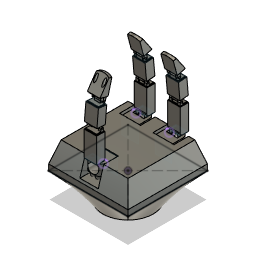
3_finger_gripper_nirmit (Autodesk Fusion 360 design; units mm, degrees)
Autodesk Fusion 360 part; units mm, degrees
note: some values were not read from the file. Chosen so that the rebuilt part matches the saved one: which face or edge a step refers to.
(part 1 of 2)
sketch "Sketch1" plane through (0, 0, 0) normal (0, 1, 0) x (1, 0, 0) in component "base v7"
  circle A0 centre (0, 0) radius 30
  dimension "d3_1" = 60
  constraint coincident A0.centre origin
  measures "d3_1" diameter of A0
ref_plane "WorkPlane1" through (0, 30, 0) normal (0, 1, 0) x (0, 0, 1) in component "base v7"
sketch "Sketch2" plane through (0, 30, 0) normal (0, 1, 0) x (1, 0, 0) in component "base v7"
  line L0 (47.5, 47.5) -> (-47.5, 47.5)
  line L1 (-47.5, 47.5) -> (-47.5, -47.5)
  line L2 (-47.5, -47.5) -> (47.5, -47.5)
  line L3 (47.5, -47.5) -> (47.5, 47.5)
  line L4 (47.5, 47.5) -> (-47.5, -47.5) construction
  line L5 (-47.5, 47.5) -> (47.5, -47.5) construction
  dimension "d6_1" = 95
  dimension "d7_1" = 95
  constraint horizontal L0
  constraint perpendicular L0 L1
  constraint parallel L0 L2
  constraint parallel L1 L3
  constraint coincident L4 origin
  constraint coincident L5 origin
  measures "d6_1" distance of L1.end L2.end
  measures "d7_1" distance of L0.start L2.end
loft "Loft1" add profiles "Sketch1", "Sketch2" section 1 section 2 makes body 1 in component "base v7"
ref_plane "WorkPlane2" through (0, 37, 0) normal (0, 1, 0) x (0, 0, 1) in component "base v7"
sketch "Sketch3" plane through (0, 37, 0) normal (0, 1, 0) x (1, 0, 0) in component "base v7"
  line L0 (47.5, -47.5) -> (-47.5, -47.5)
  line L1 (-47.5, -47.5) -> (-47.5, 47.5)
  line L2 (-47.5, 47.5) -> (47.5, 47.5)
  line L3 (47.5, 47.5) -> (47.5, -47.5)
  line L4 (47.5, -47.5) -> (-47.5, 47.5) construction
  line L5 (-47.5, -47.5) -> (47.5, 47.5) construction
  line L6 (47.5, 47.5) -> (-47.5, 47.5)
  line L7 (47.5, -47.5) -> (47.5, 47.5)
  constraint horizontal L0
  constraint perpendicular L0 L1
  constraint parallel L0 L2
  constraint parallel L1 L3
  constraint coincident L4 origin
  constraint coincident L5 origin
  constraint equal L2 L6
  constraint equal L3 L7
loft "Loft2" add profiles "Sketch2", "Sketch3" section 1 section 2 bodies 1 in component "base v7"
ref_plane "WorkPlane3" through (0, 62, 0) normal (0, 1, 0) x (0, 0, 1) in component "base v7"
sketch "Sketch4" plane through (0, 62, 0) normal (0, 1, 0) x (1, 0, 0) in component "base v7"
  line L0 (40, -40) -> (-40, -40)
  line L1 (-40, -40) -> (-40, 40)
  line L2 (-40, 40) -> (40, 40)
  line L3 (40, 40) -> (40, -40)
  line L4 (40, -40) -> (-40, 40) construction
  line L5 (-40, -40) -> (40, 40) construction
  dimension "d13_1" = 80
  dimension "d14_1" = 80
  constraint horizontal L0
  constraint perpendicular L0 L1
  constraint parallel L0 L2
  constraint parallel L1 L3
  constraint coincident L4 origin
  constraint coincident L5 origin
  measures "d13_1" distance of L1.end L2.end
  measures "d14_1" distance of L0.end L1.end
loft "Loft3" add profiles "Sketch4" section 1 face at (-15.8333, 37, -15.8333) section 2 on bodies 1 bodies 1 in component "base v7"
sketch "Sketch5" plane through (0, 16.1284, 53.7615) normal (0, 0.287348, 0.957826) x (1, 0, 0) in component "base v7"
  line L0 (-47.5, 21.7905) -> (47.5, 21.7905)
  line L1 (47.5, 21.7905) -> (40, 47.8913)
  line L2 (40, 47.8913) -> (-40, 47.8913)
  line L3 (-40, 47.8913) -> (-47.5, 21.7905)
  line L4 (-11, 47.8913) -> (11, 47.8913)
  line L5 (11, 47.8913) -> (11, 25.8913)
  line L6 (11, 25.8913) -> (-11, 25.8913)
  line L7 (-11, 25.8913) -> (-11, 47.8913)
  dimension "d17" = 22
  dimension "d18" = 22
  dimension "d20" = 29
  constraint horizontal L4
  constraint vertical L5
  constraint horizontal L6
  constraint vertical L7
  constraint coincident L2 L4.start
  measures "d17" distance of L4.end L5.end
  measures "d18" distance of L4.start L4.end
  measures "d20" distance of L1.end L5
ref_plane "WorkPlane4" through (0, 33.5, 22.5) normal (0, 0, 1) x (1, 0, 0) in component "base v7"
sketch "Sketch6" plane through (0, 33.5, 22.5) normal (0, 0, 1) x (1, 0, 0) in component "base v7"
  line L0 (-11, 28.5) -> (11, 28.5)
  line L1 (11, 28.5) -> (11, 6.5)
  line L2 (11, 6.5) -> (-11, 6.5)
  line L3 (-11, 6.5) -> (-11, 28.5)
  point P0 (-11, 28.5)
  point P1 (40, 28.5)
  dimension "d23" = 22
  dimension "d24" = 22
  dimension "d25" = 29
  constraint horizontal L0
  constraint vertical L1
  constraint horizontal L2
  constraint vertical L3
  constraint coincident L0 P0
  measures "d23" distance of P0 L2.end
  measures "d24" distance of P0 L0.end
  measures "d25" distance of L1 P1
extrude "Extrude1" cut sketch "Sketch6" along normal through all bodies 1 in component "base v7"
sketch "Sketch7" plane through (0, 0, 22.5) normal (0, 0, 1) x (1, 0, 0) in component "base v7"
  line L0 (-11, 40) -> (11, 40)
  line L1 (11, 40) -> (11, 62)
  line L2 (11, 62) -> (-11, 62)
  line L3 (-11, 62) -> (-11, 40)
  circle A0 centre (0, 51) radius 1.5
  dimension "d29" = 3
  dimension "d30" = 11
  dimension "d31" = 11
  measures "d29" diameter of A0
  measures "d30" distance of L2 A0.centre
  measures "d31" distance of L1 A0.centre
extrude "Extrude2" cut sketch "Sketch7" against normal blind 3 contours A0 bodies 1 in component "base v7"
ref_plane "WorkPlane5" through (0, 33.5, -22.5) normal (0, 0, -1) x (-1, 0, 0) in component "base v7"
sketch "Sketch8" plane through (0, 33.5, -22.5) normal (0, 0, -1) x (1, 0, 0) in component "base v7"
  line L0 (32.5, -28.5) -> (7.5, -28.5)
  line L1 (7.5, -28.5) -> (7.5, -6.5)
  line L2 (7.5, -6.5) -> (32.5, -6.5)
  line L3 (32.5, -6.5) -> (32.5, -28.5)
  line L4 (-7.5, -28.5) -> (-32.5, -28.5)
  line L5 (-32.5, -28.5) -> (-32.5, -6.5)
  line L6 (-32.5, -6.5) -> (-7.5, -6.5)
  line L7 (-7.5, -6.5) -> (-7.5, -28.5)
  line L8 (-40, -28.5) -> (40, -28.5)
  dimension "d35" = 22
  dimension "d36" = 25
  dimension "d37" = 22
  dimension "d38" = 25
  dimension "d42" = 7.5
  dimension "d43" = 7.5
  constraint horizontal L0
  constraint vertical L1
  constraint horizontal L2
  constraint vertical L3
  constraint horizontal L4
  constraint vertical L5
  constraint horizontal L6
  constraint vertical L7
  constraint coincident L0.start L8
  constraint coincident L4.start L8
  measures "d35" distance of L0.start L2.end
  measures "d36" distance of L0.start L0.end
  measures "d37" distance of L4.end L5.end
  measures "d38" distance of L4.start L4.end
  measures "d42" distance of L3 L8.end
  measures "d43" distance of L5 L8.start
extrude "Extrude3" cut sketch "Sketch8" along normal through all bodies 1 in component "base v7"
sketch "Sketch9" plane through (0, 0, -22.5) normal (0, 0, -1) x (-1, 0, 0) in component "base v7"
  line L0 (-7.5, 62) -> (-32.5, 62)
  line L1 (-32.5, 62) -> (-32.5, 40)
  line L2 (-32.5, 40) -> (-7.5, 40)
  line L3 (-7.5, 40) -> (-7.5, 62)
  circle A0 centre (-20, 51) radius 1.5
  circle A1 centre (20, 51) radius 1.5
  line L4 (7.5, 40) -> (7.5, 62)
  line L5 (7.5, 62) -> (32.5, 62)
  dimension "d45" = 3
  dimension "d46" = 11
  dimension "d47" = 12.5
  dimension "d48" = 3
  dimension "d49" = 12.5
  dimension "d50" = 11
  measures "d45" diameter of A0
  measures "d46" distance of L0 A0.centre
  measures "d47" distance of L1 A0.centre
  measures "d48" diameter of A1
  measures "d49" distance of A1.centre L4
  measures "d50" distance of A1.centre L5
extrude "Extrude4" cut sketch "Sketch9" against normal blind 3 contours A0 | A1 bodies 1 in component "base v7"
sketch "Sketch1 (2)" plane through (0, 0, 0) normal (1, 0, 0) x (0, 0, -1) in component "top v5"
  line L0 (0, 0) -> (20, 0)
  line L1 (20, 0) -> (20, 10)
  line L2 (20, 10) -> (0, 3)
  line L3 (0, 3) -> (0, 0)
  dimension "d5_3" = 20
  dimension "d6_3" = 10
  dimension "d7_3" = 3
  constraint coincident L0.start L3.end
  constraint horizontal L0
  constraint perpendicular L0 L1
  constraint perpendicular L0 L3
  measures "d5_3" distance of L0.start L0.end
  measures "d6_3" distance of L0.end L1.end
  measures "d7_3" distance of L2.end L0.start
extrude "Extrude1'" add sketch "Sketch1 (2)" along normal blind 15 separate body makes body 2 in component "top v5"
sketch "Sketch2 (2)" plane through (15, 0, 0) normal (1, 0, 0) x (0, 0, -1) in component "top v5"
  line L0 (0, 3) -> (0, 0)
  line L1 (0, 0) -> (20, 0)
  line L2 (20, 0) -> (20, 10)
  line L3 (20, 10) -> (0, 3)
ref_plane "WorkPlane1" through (7.5, 5, -21) normal (0, 0, -1) x (0, 1, 0) in component "top v5"
sketch "Sketch3 (2)" plane through (7.5, 5, -21) normal (0, 0, -1) x (1, 0, 0) in component "top v5"
  line L0 (-6.5, 4) -> (6.5, 4)
  line L1 (6.5, 4) -> (6.5, -4)
  line L2 (6.5, -4) -> (-6.5, -4)
  line L3 (-6.5, -4) -> (-6.5, 4)
  line L4 (-6.5, 4) -> (6.5, -4) construction
  line L5 (6.5, 4) -> (-6.5, -4) construction
  dimension "d17_2" = 13
  dimension "d18_2" = 8
  constraint horizontal L0
  constraint perpendicular L0 L1
  constraint parallel L0 L2
  constraint parallel L1 L3
  constraint coincident L4 origin
  constraint coincident L5 origin
  measures "d17_2" distance of L1.end L2.end
  measures "d18_2" distance of L0.start L2.end
extrude "Extrude2'" add sketch "Sketch3 (2)" against normal blind 1 bodies 2 in component "top v5"
sketch "Sketch4 (2)" plane through (14, 0, 0) normal (1, 0, 0) x (0, 0, -1) in component "top v5"
  line L0 (21, 1) -> (21, 9)
  line L1 (21, 9) -> (20, 9)
  line L2 (20, 9) -> (20, 1)
  line L3 (20, 1) -> (21, 1)
  line L4 (21, 2.5) -> (25, 2.5) construction
  circle A0 centre (25, 2.5) radius 1.5
  line L5 (0, 0) -> (20, 0)
  circle A1 centre (25, 2.5) radius 1
  line L6 (21, 4) -> (25, 4)
  line L7 (21, 1) -> (25, 1)
  dimension "d22_1" = 3
  dimension "d24_1" = 4
  dimension "d26_2" = 2
  dimension "d27_1" = 1.5
  constraint coincident L0 L4.start
  constraint perpendicular L0 L4
  constraint coincident L4.end A0.centre
  constraint concentric A0 A1
  constraint coincident L0 L6.start
  constraint perpendicular L0 L6
  constraint tangent A0 L6
  constraint horizontal L7
  constraint tangent A0 L7
  constraint coincident A0 L6.end
  constraint coincident L0.start L3.end
  constraint coincident A0 L7.end
  measures "d22_1" diameter of A0
  measures "d24_1" distance of L4.start L4.end
  measures "d26_2" diameter of A1
  measures "d27_1" distance of L3 L4
extrude "Extrude3'" add sketch "Sketch4 (2)" against normal blind 3 contours L0 A0 L6 L7 | A0 bodies 2 in component "top v5"
sketch "Sketch5 (2)" plane through (1, 0, 0) normal (-1, 0, 0) x (0, 0, 1) in component "top v5"
  line L0 (-21, 9) -> (-21, 1)
  line L1 (-21, 1) -> (-20, 1)
  line L2 (-20, 1) -> (-20, 9)
  line L3 (-20, 9) -> (-21, 9)
  circle A0 centre (-25, 2.5) radius 1.5
  circle A1 centre (-25, 2.5) radius 1
  line L4 (-25, 4) -> (-21, 4)
  line L5 (-21, 1) -> (-25, 1)
  line L6 (-21, 2.5) -> (-25, 2.5) construction
  point P0 (-25, 2.5)
  dimension "d31_1" = 3
  dimension "d32_1" = 2
  dimension "d33_1" = 3
  dimension "d34_1" = 4
  constraint concentric A0 A1
  constraint coincident L0 L4.end
  constraint perpendicular L0 L4
  constraint coincident L0.end L1.start
  constraint perpendicular L0 L5
  constraint coincident A0 L5.end
  constraint tangent A0 L4
  constraint coincident A0 L4.start
  constraint coincident L0 L6.start
  constraint coincident P0 A0.centre
  constraint coincident L6 P0
  measures "d31_1" diameter of A0
  measures "d32_1" diameter of A1
  measures "d33_1" distance of L4 L5
  measures "d34_1" distance of L6.start P0
extrude "Extrude4'" add sketch "Sketch5 (2)" against normal blind 3 contours L0 A0 L4 L5 | A0 bodies 2 in component "top v5"
sketch "Sketch6 (2)" plane through (0, 0, 0) normal (0, -1, 0) x (1, 0, 0) in component "top v5"
  line L0 (0, 0) -> (0, -20)
  line L1 (0, -20) -> (15, -20)
  line L2 (15, -20) -> (15, 0)
  line L3 (15, 0) -> (0, 0)
sketch "Sketch7 (2)" plane through (0, 0, -21) normal (0, 0, -1) x (-1, 0, 0) in component "top v5"
  line L0 (-4, 4) -> (-1, 4)
  line L1 (-1, 4) -> (-1, 9)
  line L2 (-1, 9) -> (-14, 9)
  line L3 (-14, 9) -> (-14, 4)
  line L4 (-14, 4) -> (-11, 4)
  line L5 (-11, 4) -> (-11, 1)
  line L6 (-11, 1) -> (-4, 1)
  line L7 (-4, 1) -> (-4, 4)
sketch "Sketch8 (2)" plane through (0, 0, -21) normal (0, 0, -1) x (-1, 0, 0) in component "top v5"
sketch "Sketch9 (2)" plane through (0, 0, 0) normal (0, 0, 1) x (1, 0, 0) in component "top v5"
  line L0 (0, 3) -> (0, 0)
  line L1 (0, 0) -> (15, 0)
  line L2 (15, 0) -> (15, 3)
  line L3 (15, 3) -> (0, 3)
  circle A0 centre (2.5, 5.5) radius 1.5
  line L4 (0, 10) -> (0, 3)
  line L5 (7.5, 3) -> (7.5, 9.6608) construction
  circle A1 centre (12.5, 5.5) radius 1.5
  dimension "d41" = 3
  dimension "d42_1" = 2.5
  dimension "d43_1" = 2.5
  constraint midpoint L3 L5.start
  constraint perpendicular L3 L5
  constraint symmetric A0 L5 A1
  measures "d41" diameter of A0
  measures "d42_1" distance of L3 A0.centre
  measures "d43_1" distance of A0.centre L4
extrude "Extrude5" cut sketch "Sketch9 (2)" against normal blind 15 contours A0 | A1 bodies 2 in component "top v5"
sketch "Sketch10" plane through (0, 0, 0) normal (0, -1, 0) x (1, 0, 0) in component "top v5"
sketch "Sketch11" plane through (0, 0, 0) normal (0, -1, 0) x (1, 0, 0) in component "top v5"
sketch "Sketch12" plane through (0, 0, 0) normal (0, -1, 0) x (1, 0, 0) in component "top v5"
  line L0 (0, 0) -> (0, -20)
  line L1 (0, -20) -> (15, -20)
  line L2 (15, -20) -> (15, 0)
  line L3 (15, 0) -> (0, 0)
  spline S0 degree 5 poles (0, -2) (0.5838, -1.6896) (1.7517, -1.1357) (3.5045, -0.5055) (5.8468, -0.0305) (8.8064, 0.0199) (11.2274, -0.4094) (13.0916, -1.0608) (14.3597, -1.6595) (15, -2) knots 0 0 0 0 0 0 0.2 0.4 0.6 0.8 1 1 1 1 1 1
  line L4 (13.4574, -1.1798) -> (16.5426, -2.8202)
  line L5 (15, -20) -> (15, 0)
  line L6 (-1.4063, -2.7478) -> (1.4063, -1.2522)
  line L7 (0, 0) -> (0, -20)
  line L8 (0, -2) -> (0, 0)
  line L9 (15, 0) -> (15, -2)
  dimension "d46_1" = 62
  dimension "d47_1" = 62
  dimension "d53" = 2
  dimension "d54" = 2
  constraint coincident L0 S0.start
  constraint coincident L2 S0.end
  constraint midpoint S0.end L4
  constraint midpoint S0.start L6
  constraint coincident L0.start L3.end
  constraint coincident L2.end L3.start
  measures "d46_1" angle of L4 L5
  measures "d47_1" angle of L6 L7
  measures "d53" distance of L0.start S0.start
  measures "d54" distance of S0.end L2.end
extrude "Extrude6" cut sketch "Sketch12" against normal through all contours L0 L2 L3 S0 L5 L7 L8 L9 bodies 2 in component "top v5"
sketch "Sketch1 (3)" plane through (0, 0, 0) normal (0, 1, 0) x (1, 0, 0) in component "middle v4"
  line L0 (7.5, -10) -> (-7.5, -10)
  line L1 (-7.5, -10) -> (-7.5, 10)
  line L2 (-7.5, 10) -> (7.5, 10)
  line L3 (7.5, 10) -> (7.5, -10)
  line L4 (7.5, -10) -> (-7.5, 10) construction
  line L5 (-7.5, -10) -> (7.5, 10) construction
  dimension "d4_2" = 15
  dimension "d5_4" = 20
  constraint horizontal L0
  constraint perpendicular L0 L1
  constraint parallel L0 L2
  constraint parallel L1 L3
  constraint coincident L4 origin
  constraint coincident L5 origin
  measures "d4_2" distance of L1.end L2.end
  measures "d5_4" distance of L0.start L2.end
extrude "Extrude1''" add sketch "Sketch1 (3)" along normal blind 10 separate body makes body 3 in component "middle v4"
sketch "Sketch2 (3)" plane through (0, 0, -10) normal (0, 0, -1) x (-1, 0, 0) in component "middle v4"
  line L0 (-7.5, 0) -> (7.5, 0)
  line L1 (7.5, 0) -> (7.5, 10)
  line L2 (7.5, 10) -> (-7.5, 10)
  line L3 (-7.5, 10) -> (-7.5, 0)
sketch "Sketch3 (3)" plane through (0, 0, -10) normal (0, 0, -1) x (-1, 0, 0) in component "middle v4"
  line L0 (-6.5, 9) -> (6.5, 9)
  line L1 (6.5, 9) -> (6.5, 1)
  line L2 (6.5, 1) -> (-6.5, 1)
  line L3 (-6.5, 1) -> (-6.5, 9)
  line L4 (7.5, 10) -> (-7.5, 10)
  line L5 (-7.5, 10) -> (-7.5, 0)
  dimension "d11_1" = 8
  dimension "d12_2" = 13
  dimension "d13_2" = 1
  dimension "d14_2" = 1
  constraint horizontal L0
  constraint vertical L1
  constraint horizontal L2
  constraint vertical L3
  measures "d11_1" distance of L0.end L1.end
  measures "d12_2" distance of L0.start L0.end
  measures "d13_2" distance of L0 L4
  measures "d14_2" distance of L3 L5
extrude "Extrude2''" add sketch "Sketch3 (3)" along normal blind 1 bodies 3 in component "middle v4"
sketch "Sketch4 (3)" plane through (0, 0, -11) normal (0, 0, -1) x (-1, 0, 0) in component "middle v4"
  line L0 (-6.5, 1) -> (6.5, 1)
  line L1 (6.5, 1) -> (6.5, 9)
  line L2 (6.5, 9) -> (-6.5, 9)
  line L3 (-6.5, 9) -> (-6.5, 1)
ref_plane "WorkPlane1" through (0, 5, -10.5) normal (1, 0, 0) x (0, -1, 0) in component "middle v4"
sketch "Sketch5 (3)" plane through (0, 5, -10.5) normal (1, 0, 0) x (0, 0, -1) in component "middle v4"
sketch "Sketch6 (3)" plane through (0, 0, -11) normal (0, 0, -1) x (-1, 0, 0) in component "middle v4"
sketch "Sketch7 (3)" plane through (0, 0, -11) normal (0, 0, -1) x (-1, 0, 0) in component "middle v4"
sketch "Sketch8 (3)" plane through (0, 0, -11) normal (0, 0, -1) x (1, 0, 0) in component "middle v4"
sketch "Sketch9 (3)" plane through (0, 5, -10.5) normal (1, 0, 0) x (0, 0, -1) in component "middle v4"
sketch "Sketch10 (2)" plane through (0, 5, -10.5) normal (1, 0, 0) x (0, 0, -1) in component "middle v4"
sketch "Sketch11 (2)" plane through (0, 5, -10.5) normal (1, 0, 0) x (0, 0, -1) in component "middle v4"
  line L0 (0, 0) -> (0.5, 0) construction
  line L1 (0.5, 0) -> (0.5, -4) construction
  circle A0 centre (3, -2.5) radius 1
  circle A1 centre (3, -2.5) radius 1.5
  line L2 (0.5, -2.5) -> (3, -2.5) construction
  line L3 (0.5, -4) -> (3, -4)
  line L4 (0.5, -1) -> (3, -1)
  line L5 (0.5, -1) -> (0.5, -4)
  dimension "d18_3" = 0.5
  dimension "d19_2" = 4
  dimension "d22_2" = 3
  dimension "d23_1" = 2
  dimension "d25_2" = 2.5
  constraint coincident L0.start origin
  constraint horizontal L0
  constraint perpendicular L0 L1
  constraint concentric A0 A1
  constraint coincident L1 L2.start
  constraint perpendicular L1 L2
  constraint coincident A0.centre A1.centre
  constraint perpendicular L1 L3
  constraint tangent A1 L3
  constraint coincident A1 L3.end
  constraint coincident L1 L4.start
  constraint perpendicular L1 L4
  constraint tangent A1 L4
  constraint coincident A1 L4.end
  measures "d18_3" distance of L0.start L0.end
  measures "d19_2" distance of L0.end L1.end
  measures "d22_2" diameter of A1
  measures "d23_1" diameter of A0
  measures "d25_2" distance of L2.start A0.centre
sketch "Sketch12 (2)" plane through (0, 5, -10.5) normal (1, 0, 0) x (0, 0, -1) in component "middle v4"
extrude "Extrude3''" add sketch "Sketch11 (2)" along normal blind 3.5 and the other way blind 3.5 bodies 3 in component "middle v4"
ref_plane "WorkPlane2" through (0, 5, 0) normal (0, 0, 1) x (1, 0, 0) in component "middle v4"
mirror "Mirror1" about plane through (0, 5, 0) normal (0, 0, 1) of "Extrude2''", "Extrude3''" in component "middle v4"
sketch "Sketch1 (4)" plane through (0, 0, 0) normal (0, 1, 0) x (1, 0, 0) in component "end v6"
  line L0 (7.5, -15) -> (-7.5, -15)
  line L1 (-7.5, -15) -> (-7.5, 15)
  line L2 (-7.5, 15) -> (7.5, 15)
  line L3 (7.5, 15) -> (7.5, -15)
  line L4 (7.5, -15) -> (-7.5, 15) construction
  line L5 (-7.5, -15) -> (7.5, 15) construction
  dimension "d4_3" = 30
  dimension "d5_5" = 15
  constraint horizontal L0
  constraint perpendicular L0 L1
  constraint parallel L0 L2
  constraint parallel L1 L3
  constraint coincident L4 origin
  constraint coincident L5 origin
  measures "d4_3" distance of L0.start L2.end
  measures "d5_5" distance of L0.start L0.end
extrude "Extrude1'''" add sketch "Sketch1 (4)" along normal blind 10 separate body makes body 4 in component "end v6"
sketch "Sketch2 (4)" plane through (0, 0, -15) normal (0, 0, -1) x (-1, 0, 0) in component "end v6"
  line L0 (-7.5, 0) -> (7.5, 0)
  line L1 (7.5, 0) -> (7.5, 10)
  line L2 (7.5, 10) -> (-7.5, 10)
  line L3 (-7.5, 10) -> (-7.5, 0)
  line L4 (-6.5, 9) -> (6.5, 9)
  line L5 (6.5, 9) -> (6.5, 1)
  line L6 (6.5, 1) -> (-6.5, 1)
  line L7 (-6.5, 1) -> (-6.5, 9)
  dimension "d10_1" = 13
  dimension "d11_2" = 8
  dimension "d12_3" = 1
  dimension "d13_3" = 1
  constraint horizontal L4
  constraint vertical L5
  constraint horizontal L6
  constraint vertical L7
  measures "d10_1" distance of L4.start L4.end
  measures "d11_2" distance of L4.end L5.end
  measures "d12_3" distance of L2 L4
  measures "d13_3" distance of L3 L7
extrude "Extrude2'''" add sketch "Sketch2 (4)" along normal blind 1 contours L4 L5 L6 L7 bodies 4 in component "end v6"
ref_plane "WorkPlane1" through (0, 5, -15.5) normal (1, 0, 0) x (0, -1, 0) in component "end v6"
sketch "Sketch3 (4)" plane through (6.5, 0, 0) normal (1, 0, 0) x (0, 0, -1) in component "end v6"
  line L0 (15, 9) -> (15, 1)
  line L1 (15, 1) -> (16, 1)
  line L2 (16, 1) -> (16, 9)
  line L3 (16, 9) -> (15, 9)
  line L4 (16, 1) -> (18.5, 1)
  line L5 (16, 2.5) -> (18.5, 2.5) construction
  circle A0 centre (18.5, 2.5) radius 1.5
  circle A1 centre (18.5, 2.5) radius 1
  line L6 (16, 4) -> (18.5, 4)
  dimension "d20_3" = 2.5
  dimension "d21" = 3
  dimension "d22_3" = 2
  constraint coincident L1.end L2.start
  constraint perpendicular L2 L4
  constraint coincident L2 L5.start
  constraint perpendicular L2 L5
  constraint coincident L5.end A0.centre
  constraint concentric A0 A1
  constraint coincident L2 L6.start
  constraint perpendicular L2 L6
  constraint tangent L4 A0
  constraint tangent A0 L6
  constraint coincident A0 L6.end
  constraint coincident L4.end A0
  measures "d20_3" distance of L5.start L5.end
  measures "d21" diameter of A0
  measures "d22_3" diameter of A1
extrude "Extrude3'''" add sketch "Sketch3 (4)" against normal blind 3 contours L2 L4 A0 L6 | A0 bodies 4 in component "end v6"
mirror "Mirror1'" about plane through (0, 5, -15.5) normal (1, 0, 0) of "Extrude2'''", "Extrude3'''" in component "end v6"
ref_plane "WorkPlane2" through (0, 5, 0) normal (0, 0, 1) x (1, 0, 0) in component "end v6"
mirror "Mirror2" about plane through (0, 5, 0) normal (0, 0, 1) of 13 faces at (3.5, 2.5, -16.5) (4.5, 3.4925, -19.6247) (5.5, 4, -16.8333) (-4.5, 3.5474, -19.5738) (-6.5, 2.5, -16.1667) (-5.5, 4, -16.8333) (1.1667, 7.3333, -16) (6.5, 2.5, -16.1667) (2.1667, 9, -15.3333) (5.5, 1, -16.5) (-3.5, 2.5, -16.5) (5.5, 2.4004, -19.495) (-5.5, 2.4004, -19.495) on bodies 4 in component "end v6"
sketch "Sketch4 (4)" plane through (0, 0, 15) normal (0, 0, 1) x (1, 0, 0) in component "end v6"
  line L0 (6.5, 9) -> (6.5, 1)
  line L1 (6.5, 1) -> (-6.5, 1)
  line L2 (-6.5, 1) -> (-6.5, 9)
  line L3 (-6.5, 9) -> (6.5, 9)
  line L4 (-7.5, 0) -> (7.5, 0)
  line L5 (7.5, 0) -> (7.5, 10)
  line L6 (7.5, 10) -> (-7.5, 10)
  line L7 (-7.5, 10) -> (-7.5, 0)
sketch "Sketch5 (4)" plane through (6.5, 0, 0) normal (1, 0, 0) x (0, 0, -1) in component "end v6"
  circle A0 centre (-18.5, 2.5) radius 1
  line L0 (-16, 9) -> (-16, 4)
  line L1 (-16, 4) -> (-18.5, 4)
  arc A1 (-18.5, 4) -> (-18.5, 1) centre (-18.5, 2.5) ccw
  line L2 (-18.5, 1) -> (-15, 1)
  line L3 (-15, 1) -> (-15, 9)
  line L4 (-15, 9) -> (-16, 9)
sketch "Sketch6 (4)" plane through (0, 0, 16) normal (0, 0, 1) x (1, 0, 0) in component "end v6"
  line L0 (-3.5, 4) -> (-3.5, 1)
  line L1 (-3.5, 1) -> (3.5, 1)
  line L2 (3.5, 1) -> (3.5, 4)
  line L3 (3.5, 4) -> (6.5, 4)
  line L4 (6.5, 4) -> (6.5, 9)
  line L5 (6.5, 9) -> (-6.5, 9)
  line L6 (-6.5, 9) -> (-6.5, 4)
  line L7 (-6.5, 4) -> (-3.5, 4)
fillet "Fillet1" radius 3 1 edges at (0, 0, 15) on bodies 4 in component "end v6"
sketch "Sketch1 (5)" plane through (0, 0, 0) normal (1, 0, 0) x (0, 0, -1) in component "turner v14"
  line L0 (10, -10) -> (-10, -10)
  line L1 (-10, -10) -> (-10, 10)
  line L2 (-10, 10) -> (10, 10)
  line L3 (10, 10) -> (10, -10)
  line L4 (10, -10) -> (-10, 10) construction
  line L5 (-10, -10) -> (10, 10) construction
  dimension "d4_4" = 20
  dimension "d5_6" = 20
  constraint horizontal L0
  constraint perpendicular L0 L1
  constraint parallel L0 L2
  constraint parallel L1 L3
  constraint coincident L4 origin
  constraint coincident L5 origin
  measures "d4_4" distance of L0.start L2.end
  measures "d5_6" distance of L0.start L0.end
extrude "Extrude1''''" add sketch "Sketch1 (5)" along normal blind 20 separate body makes body 5 in component "turner v14"
sketch "Sketch2 (5)" plane through (0, 0, -10) normal (0, 0, -1) x (-1, 0, 0) in component "turner v14"
  line L0 (0, -10) -> (0, 10)
  line L1 (0, 10) -> (-20, 10)
  line L2 (-20, 10) -> (-20, -10)
  line L3 (-20, -10) -> (0, -10)
  line L4 (-10, 10) -> (-3.5, 10)
  line L5 (-3.5, 10) -> (-3.5, 3.5)
  line L6 (-10, 10) -> (-10, 4.4853) construction
  line L7 (-10, 10) -> (-16.5, 10)
  line L8 (-16.5, 10) -> (-16.5, 3.5)
  arc A0 (-16.5, 3.5) -> (-3.5, 3.5) centre (-10, 3.5) ccw
  dimension "d12_4" = 6.5
  dimension "d13_4" = 6.5
  constraint midpoint L1 L4.start
  constraint parallel L1 L4
  constraint perpendicular L4 L5
  constraint perpendicular L1 L6
  constraint symmetric L4.start L6 L7.start
  constraint symmetric L4.end L6 L7.end
  constraint symmetric L5.end L6 L8.end
  constraint tangent L5 A0
  measures "d12_4" distance of L4.start L4.end
  measures "d13_4" distance of L4.end L5.end
extrude "Extrude2''''" cut sketch "Sketch2 (5)" against normal blind 10 contours L1 L4 L5 L7 L8 A0 bodies 5 in component "turner v14"
sketch "Sketch3 (5)" plane through (3.5, 0, 0) normal (1, 0, 0) x (0, 0, -1) in component "turner v14"
  line L0 (10, 3.5) -> (10, 10)
  line L1 (10, 10) -> (0, 10)
  line L2 (0, 10) -> (0, 3.5)
  line L3 (0, 3.5) -> (10, 3.5)
  line L4 (5, 3.5) -> (5, 7.5) construction
  circle A0 centre (5, 7.5) radius 1
  dimension "d20_4" = 4
  dimension "d22_4" = 5
  dimension "d23_2" = 2
  constraint coincident L3 L4.start
  constraint perpendicular L3 L4
  constraint coincident L4.end A0.centre
  measures "d20_4" distance of L4.start L4.end
  measures "d22_4" distance of L0 L4
  measures "d23_2" diameter of A0
extrude "Extrude3''''" add sketch "Sketch3 (5)" along normal up to surface (13 mm away) contours A0 bodies 5 in component "turner v14"
sketch "Sketch4 (5)" plane through (0, 0, 10) normal (0, 0, 1) x (1, 0, 0) in component "turner v14"
  line L0 (0, 10) -> (0, -10)
  line L1 (0, -10) -> (20, -10)
  line L2 (20, -10) -> (20, 10)
  line L3 (20, 10) -> (0, 10)
sketch "Sketch5 (5)" plane through (0, 0, 10) normal (0, 0, 1) x (1, 0, 0) in component "turner v14"
  circle A0 centre (10, 0) radius 1.5
  line L0 (20, 10) -> (0, 10)
  line L1 (20, -10) -> (20, 10)
  dimension "d28_3" = 3
  dimension "d29_5" = 10
  dimension "d30_4" = 10
  measures "d28_3" diameter of A0
  measures "d29_5" distance of A0.centre L0
  measures "d30_4" distance of A0.centre L1
extrude "Extrude4''" add sketch "Sketch5 (5)" along normal blind 3 bodies 5 in component "turner v14"
fillet "Fillet1'" radius 7 1 edges at (10, -10, -10) on bodies 5 in component "turner v14"
fillet "Fillet2" radius 7 3 edges at (20, -10, 3.5) (20, -7.9497, -7.9497) (20, 3.5, -10) on bodies 5 in component "turner v14"
fillet "Fillet3" radius 7 3 edges at (0, 3.5, -10) (0, -7.9497, -7.9497) (0, -10, 3.5) on bodies 5 in component "turner v14"
sketch "Sketch1 (6)" plane through (0, 0, 0) normal (1, 0, 0) x (0, 0, -1) in component "top v5 (1)"
  line L0 (0, 0) -> (20, 0)
  line L1 (20, 0) -> (20, 10)
  line L2 (20, 10) -> (0, 3)
  line L3 (0, 3) -> (0, 0)
  dimension "d5_8" = 20
  dimension "d6_7" = 10
  dimension "d7_7" = 3
  constraint coincident L0.start L3.end
  constraint horizontal L0
  constraint perpendicular L0 L1
  constraint perpendicular L0 L3
  measures "d5_8" distance of L0.start L0.end
  measures "d6_7" distance of L0.end L1.end
  measures "d7_7" distance of L2.end L0.start
extrude "Extrude1'''''" add sketch "Sketch1 (6)" along normal blind 15 separate body makes body 6 in component "top v5 (1)"
sketch "Sketch2 (6)" plane through (15, 0, 0) normal (1, 0, 0) x (0, 0, -1) in component "top v5 (1)"
  line L0 (0, 3) -> (0, 0)
  line L1 (0, 0) -> (20, 0)
  line L2 (20, 0) -> (20, 10)
  line L3 (20, 10) -> (0, 3)
ref_plane "WorkPlane1" through (7.5, 5, -21) normal (0, 0, -1) x (0, 1, 0) in component "top v5 (1)"
sketch "Sketch3 (6)" plane through (7.5, 5, -21) normal (0, 0, -1) x (1, 0, 0) in component "top v5 (1)"
  line L0 (-6.5, 4) -> (6.5, 4)
  line L1 (6.5, 4) -> (6.5, -4)
  line L2 (6.5, -4) -> (-6.5, -4)
  line L3 (-6.5, -4) -> (-6.5, 4)
  line L4 (-6.5, 4) -> (6.5, -4) construction
  line L5 (6.5, 4) -> (-6.5, -4) construction
  dimension "d17_4" = 13
  dimension "d18_5" = 8
  constraint horizontal L0
  constraint perpendicular L0 L1
  constraint parallel L0 L2
  constraint parallel L1 L3
  constraint coincident L4 origin
  constraint coincident L5 origin
  measures "d17_4" distance of L1.end L2.end
  measures "d18_5" distance of L0.start L2.end
extrude "Extrude2'''''" add sketch "Sketch3 (6)" against normal blind 1 bodies 6 in component "top v5 (1)"
sketch "Sketch4 (6)" plane through (14, 0, 0) normal (1, 0, 0) x (0, 0, -1) in component "top v5 (1)"
  line L0 (21, 1) -> (21, 9)
  line L1 (21, 9) -> (20, 9)
  line L2 (20, 9) -> (20, 1)
  line L3 (20, 1) -> (21, 1)
  line L4 (21, 2.5) -> (25, 2.5) construction
  circle A0 centre (25, 2.5) radius 1.5
  line L5 (0, 0) -> (20, 0)
  circle A1 centre (25, 2.5) radius 1
  line L6 (21, 4) -> (25, 4)
  line L7 (21, 1) -> (25, 1)
  dimension "d22_5" = 3
  dimension "d24_4" = 4
  dimension "d26_5" = 2
  dimension "d27_5" = 1.5
  constraint coincident L0 L4.start
  constraint perpendicular L0 L4
  constraint coincident L4.end A0.centre
  constraint concentric A0 A1
  constraint coincident L0 L6.start
  constraint perpendicular L0 L6
  constraint tangent A0 L6
  constraint horizontal L7
  constraint tangent A0 L7
  constraint coincident A0 L6.end
  constraint coincident L0.start L3.end
  constraint coincident A0 L7.end
  measures "d22_5" diameter of A0
  measures "d24_4" distance of L4.start L4.end
  measures "d26_5" diameter of A1
  measures "d27_5" distance of L3 L4
extrude "Extrude3'''''" add sketch "Sketch4 (6)" against normal blind 3 contours L0 A0 L6 L7 | A0 bodies 6 in component "top v5 (1)"
sketch "Sketch5 (6)" plane through (1, 0, 0) normal (-1, 0, 0) x (0, 0, 1) in component "top v5 (1)"
  line L0 (-21, 9) -> (-21, 1)
  line L1 (-21, 1) -> (-20, 1)
  line L2 (-20, 1) -> (-20, 9)
  line L3 (-20, 9) -> (-21, 9)
  circle A0 centre (-25, 2.5) radius 1.5
  circle A1 centre (-25, 2.5) radius 1
  line L4 (-25, 4) -> (-21, 4)
  line L5 (-21, 1) -> (-25, 1)
  line L6 (-21, 2.5) -> (-25, 2.5) construction
  point P0 (-25, 2.5)
  dimension "d31_5" = 3
  dimension "d32_5" = 2
  dimension "d33_2" = 3
  dimension "d34_2" = 4
  constraint concentric A0 A1
  constraint coincident L0 L4.end
  constraint perpendicular L0 L4
  constraint coincident L0.end L1.start
  constraint perpendicular L0 L5
  constraint coincident A0 L5.end
  constraint tangent A0 L4
  constraint coincident A0 L4.start
  constraint coincident L0 L6.start
  constraint coincident P0 A0.centre
  constraint coincident L6 P0
  measures "d31_5" diameter of A0
  measures "d32_5" diameter of A1
  measures "d33_2" distance of L4 L5
  measures "d34_2" distance of L6.start P0
extrude "Extrude4'''" add sketch "Sketch5 (6)" against normal blind 3 contours L0 A0 L4 L5 | A0 bodies 6 in component "top v5 (1)"
sketch "Sketch6 (5)" plane through (0, 0, 0) normal (0, -1, 0) x (1, 0, 0) in component "top v5 (1)"
  line L0 (0, 0) -> (0, -20)
  line L1 (0, -20) -> (15, -20)
  line L2 (15, -20) -> (15, 0)
  line L3 (15, 0) -> (0, 0)
sketch "Sketch7 (4)" plane through (0, 0, -21) normal (0, 0, -1) x (-1, 0, 0) in component "top v5 (1)"
  line L0 (-4, 4) -> (-1, 4)
  line L1 (-1, 4) -> (-1, 9)
  line L2 (-1, 9) -> (-14, 9)
  line L3 (-14, 9) -> (-14, 4)
  line L4 (-14, 4) -> (-11, 4)
  line L5 (-11, 4) -> (-11, 1)
  line L6 (-11, 1) -> (-4, 1)
  line L7 (-4, 1) -> (-4, 4)
sketch "Sketch8 (4)" plane through (0, 0, -21) normal (0, 0, -1) x (-1, 0, 0) in component "top v5 (1)"
sketch "Sketch9 (4)" plane through (0, 0, 0) normal (0, 0, 1) x (1, 0, 0) in component "top v5 (1)"
  line L0 (0, 3) -> (0, 0)
  line L1 (0, 0) -> (15, 0)
  line L2 (15, 0) -> (15, 3)
  line L3 (15, 3) -> (0, 3)
  circle A0 centre (2.5, 5.5) radius 1.5
  line L4 (0, 10) -> (0, 3)
  line L5 (7.5, 3) -> (7.5, 9.6608) construction
  circle A1 centre (12.5, 5.5) radius 1.5
  dimension "d41_1" = 3
  dimension "d42_2" = 2.5
  dimension "d43_2" = 2.5
  constraint midpoint L3 L5.start
  constraint perpendicular L3 L5
  constraint symmetric A0 L5 A1
  measures "d41_1" diameter of A0
  measures "d42_2" distance of L3 A0.centre
  measures "d43_2" distance of A0.centre L4
extrude "Extrude5'" cut sketch "Sketch9 (4)" against normal blind 15 contours A0 | A1 bodies 6 in component "top v5 (1)"
sketch "Sketch10 (3)" plane through (0, 0, 0) normal (0, -1, 0) x (1, 0, 0) in component "top v5 (1)"
sketch "Sketch11 (3)" plane through (0, 0, 0) normal (0, -1, 0) x (1, 0, 0) in component "top v5 (1)"
sketch "Sketch12 (3)" plane through (0, 0, 0) normal (0, -1, 0) x (1, 0, 0) in component "top v5 (1)"
  line L0 (0, 0) -> (0, -20)
  line L1 (0, -20) -> (15, -20)
  line L2 (15, -20) -> (15, 0)
  line L3 (15, 0) -> (0, 0)
  spline S0 degree 5 poles (0, -2) (0.5838, -1.6896) (1.7517, -1.1357) (3.5045, -0.5055) (5.8468, -0.0305) (8.8064, 0.0199) (11.2274, -0.4094) (13.0916, -1.0608) (14.3597, -1.6595) (15, -2) knots 0 0 0 0 0 0 0.2 0.4 0.6 0.8 1 1 1 1 1 1
  line L4 (13.4574, -1.1798) -> (16.5426, -2.8202)
  line L5 (15, -20) -> (15, 0)
  line L6 (-1.4063, -2.7478) -> (1.4063, -1.2522)
  line L7 (0, 0) -> (0, -20)
  line L8 (0, -2) -> (0, 0)
  line L9 (15, 0) -> (15, -2)
  dimension "d46_2" = 62
  dimension "d47_2" = 62
  dimension "d53_1" = 2
  dimension "d54_1" = 2
  constraint coincident L0 S0.start
  constraint coincident L2 S0.end
  constraint midpoint S0.end L4
  constraint midpoint S0.start L6
  constraint coincident L0.start L3.end
  constraint coincident L2.end L3.start
  measures "d46_2" angle of L4 L5
  measures "d47_2" angle of L6 L7
  measures "d53_1" distance of L0.start S0.start
  measures "d54_1" distance of S0.end L2.end
extrude "Extrude6'" cut sketch "Sketch12 (3)" against normal through all contours L0 L2 L3 S0 L5 L7 L8 L9 bodies 6 in component "top v5 (1)"
sketch "Sketch1 (7)" plane through (0, 0, 0) normal (0, 1, 0) x (1, 0, 0) in component "middle v4 (1)"
  line L0 (7.5, -10) -> (-7.5, -10)
  line L1 (-7.5, -10) -> (-7.5, 10)
  line L2 (-7.5, 10) -> (7.5, 10)
  line L3 (7.5, 10) -> (7.5, -10)
  line L4 (7.5, -10) -> (-7.5, 10) construction
  line L5 (-7.5, -10) -> (7.5, 10) construction
  dimension "d4_6" = 15
  dimension "d5_9" = 20
  constraint horizontal L0
  constraint perpendicular L0 L1
  constraint parallel L0 L2
  constraint parallel L1 L3
  constraint coincident L4 origin
  constraint coincident L5 origin
  measures "d4_6" distance of L1.end L2.end
  measures "d5_9" distance of L0.start L2.end
extrude "Extrude1''''''" add sketch "Sketch1 (7)" along normal blind 10 separate body makes body 7 in component "middle v4 (1)"
sketch "Sketch2 (7)" plane through (0, 0, -10) normal (0, 0, -1) x (-1, 0, 0) in component "middle v4 (1)"
  line L0 (-7.5, 0) -> (7.5, 0)
  line L1 (7.5, 0) -> (7.5, 10)
  line L2 (7.5, 10) -> (-7.5, 10)
  line L3 (-7.5, 10) -> (-7.5, 0)
sketch "Sketch3 (7)" plane through (0, 0, -10) normal (0, 0, -1) x (-1, 0, 0) in component "middle v4 (1)"
  line L0 (-6.5, 9) -> (6.5, 9)
  line L1 (6.5, 9) -> (6.5, 1)
  line L2 (6.5, 1) -> (-6.5, 1)
  line L3 (-6.5, 1) -> (-6.5, 9)
  line L4 (7.5, 10) -> (-7.5, 10)
  line L5 (-7.5, 10) -> (-7.5, 0)
  dimension "d11_3" = 8
  dimension "d12_5" = 13
  dimension "d13_5" = 1
  dimension "d14_3" = 1
  constraint horizontal L0
  constraint vertical L1
  constraint horizontal L2
  constraint vertical L3
  measures "d11_3" distance of L0.end L1.end
  measures "d12_5" distance of L0.start L0.end
  measures "d13_5" distance of L0 L4
  measures "d14_3" distance of L3 L5
extrude "Extrude2''''''" add sketch "Sketch3 (7)" along normal blind 1 bodies 7 in component "middle v4 (1)"
sketch "Sketch4 (7)" plane through (0, 0, -11) normal (0, 0, -1) x (-1, 0, 0) in component "middle v4 (1)"
  line L0 (-6.5, 1) -> (6.5, 1)
  line L1 (6.5, 1) -> (6.5, 9)
  line L2 (6.5, 9) -> (-6.5, 9)
  line L3 (-6.5, 9) -> (-6.5, 1)
ref_plane "WorkPlane1" through (0, 5, -10.5) normal (1, 0, 0) x (0, -1, 0) in component "middle v4 (1)"
sketch "Sketch5 (7)" plane through (0, 5, -10.5) normal (1, 0, 0) x (0, 0, -1) in component "middle v4 (1)"
sketch "Sketch6 (6)" plane through (0, 0, -11) normal (0, 0, -1) x (-1, 0, 0) in component "middle v4 (1)"
sketch "Sketch7 (5)" plane through (0, 0, -11) normal (0, 0, -1) x (-1, 0, 0) in component "middle v4 (1)"
sketch "Sketch8 (5)" plane through (0, 0, -11) normal (0, 0, -1) x (1, 0, 0) in component "middle v4 (1)"
sketch "Sketch9 (5)" plane through (0, 5, -10.5) normal (1, 0, 0) x (0, 0, -1) in component "middle v4 (1)"
sketch "Sketch10 (4)" plane through (0, 5, -10.5) normal (1, 0, 0) x (0, 0, -1) in component "middle v4 (1)"
sketch "Sketch11 (4)" plane through (0, 5, -10.5) normal (1, 0, 0) x (0, 0, -1) in component "middle v4 (1)"
  line L0 (0, 0) -> (0.5, 0) construction
  line L1 (0.5, 0) -> (0.5, -4) construction
  circle A0 centre (3, -2.5) radius 1
  circle A1 centre (3, -2.5) radius 1.5
  line L2 (0.5, -2.5) -> (3, -2.5) construction
  line L3 (0.5, -4) -> (3, -4)
  line L4 (0.5, -1) -> (3, -1)
  line L5 (0.5, -1) -> (0.5, -4)
  dimension "d18_6" = 0.5
  dimension "d19_5" = 4
  dimension "d22_6" = 3
  dimension "d23_3" = 2
  dimension "d25_6" = 2.5
  constraint coincident L0.start origin
  constraint horizontal L0
  constraint perpendicular L0 L1
  constraint concentric A0 A1
  constraint coincident L1 L2.start
  constraint perpendicular L1 L2
  constraint coincident A0.centre A1.centre
  constraint perpendicular L1 L3
  constraint tangent A1 L3
  constraint coincident A1 L3.end
  constraint coincident L1 L4.start
  constraint perpendicular L1 L4
  constraint tangent A1 L4
  constraint coincident A1 L4.end
  measures "d18_6" distance of L0.start L0.end
  measures "d19_5" distance of L0.end L1.end
  measures "d22_6" diameter of A1
  measures "d23_3" diameter of A0
  measures "d25_6" distance of L2.start A0.centre
sketch "Sketch12 (4)" plane through (0, 5, -10.5) normal (1, 0, 0) x (0, 0, -1) in component "middle v4 (1)"
extrude "Extrude3''''''" add sketch "Sketch11 (4)" along normal blind 3.5 and the other way blind 3.5 bodies 7 in component "middle v4 (1)"
ref_plane "WorkPlane2" through (0, 5, 0) normal (0, 0, 1) x (1, 0, 0) in component "middle v4 (1)"
mirror "Mirror1''" about plane through (0, 5, 0) normal (0, 0, 1) of "Extrude2''''''", "Extrude3''''''" in component "middle v4 (1)"
sketch "Sketch1 (8)" plane through (0, 0, 0) normal (0, 1, 0) x (1, 0, 0) in component "end v6 (1)"
  line L0 (7.5, -15) -> (-7.5, -15)
  line L1 (-7.5, -15) -> (-7.5, 15)
  line L2 (-7.5, 15) -> (7.5, 15)
  line L3 (7.5, 15) -> (7.5, -15)
  line L4 (7.5, -15) -> (-7.5, 15) construction
  line L5 (-7.5, -15) -> (7.5, 15) construction
  dimension "d4_7" = 30
  dimension "d5_10" = 15
  constraint horizontal L0
  constraint perpendicular L0 L1
  constraint parallel L0 L2
  constraint parallel L1 L3
  constraint coincident L4 origin
  constraint coincident L5 origin
  measures "d4_7" distance of L0.start L2.end
  measures "d5_10" distance of L0.start L0.end
extrude "Extrude1'''''''" add sketch "Sketch1 (8)" along normal blind 10 separate body makes body 8 in component "end v6 (1)"
sketch "Sketch2 (8)" plane through (0, 0, -15) normal (0, 0, -1) x (-1, 0, 0) in component "end v6 (1)"
  line L0 (-7.5, 0) -> (7.5, 0)
  line L1 (7.5, 0) -> (7.5, 10)
  line L2 (7.5, 10) -> (-7.5, 10)
  line L3 (-7.5, 10) -> (-7.5, 0)
  line L4 (-6.5, 9) -> (6.5, 9)
  line L5 (6.5, 9) -> (6.5, 1)
  line L6 (6.5, 1) -> (-6.5, 1)
  line L7 (-6.5, 1) -> (-6.5, 9)
  dimension "d10_2" = 13
  dimension "d11_4" = 8
  dimension "d12_6" = 1
  dimension "d13_6" = 1
  constraint horizontal L4
  constraint vertical L5
  constraint horizontal L6
  constraint vertical L7
  measures "d10_2" distance of L4.start L4.end
  measures "d11_4" distance of L4.end L5.end
  measures "d12_6" distance of L2 L4
  measures "d13_6" distance of L3 L7
extrude "Extrude2'''''''" add sketch "Sketch2 (8)" along normal blind 1 contours L4 L5 L6 L7 bodies 8 in component "end v6 (1)"
ref_plane "WorkPlane1" through (0, 5, -15.5) normal (1, 0, 0) x (0, -1, 0) in component "end v6 (1)"
sketch "Sketch3 (8)" plane through (6.5, 0, 0) normal (1, 0, 0) x (0, 0, -1) in component "end v6 (1)"
  line L0 (15, 9) -> (15, 1)
  line L1 (15, 1) -> (16, 1)
  line L2 (16, 1) -> (16, 9)
  line L3 (16, 9) -> (15, 9)
  line L4 (16, 1) -> (18.5, 1)
  line L5 (16, 2.5) -> (18.5, 2.5) construction
  circle A0 centre (18.5, 2.5) radius 1.5
  circle A1 centre (18.5, 2.5) radius 1
  line L6 (16, 4) -> (18.5, 4)
  dimension "d20_7" = 2.5
  dimension "d21_1" = 3
  dimension "d22_7" = 2
  constraint coincident L1.end L2.start
  constraint perpendicular L2 L4
  constraint coincident L2 L5.start
  constraint perpendicular L2 L5
  constraint coincident L5.end A0.centre
  constraint concentric A0 A1
  constraint coincident L2 L6.start
  constraint perpendicular L2 L6
  constraint tangent L4 A0
  constraint tangent A0 L6
  constraint coincident A0 L6.end
  constraint coincident L4.end A0
  measures "d20_7" distance of L5.start L5.end
  measures "d21_1" diameter of A0
  measures "d22_7" diameter of A1
extrude "Extrude3'''''''" add sketch "Sketch3 (8)" against normal blind 3 contours L2 L4 A0 L6 | A0 bodies 8 in component "end v6 (1)"
mirror "Mirror1'''" about plane through (0, 5, -15.5) normal (1, 0, 0) of "Extrude2'''''''", "Extrude3'''''''" in component "end v6 (1)"
ref_plane "WorkPlane2" through (0, 5, 0) normal (0, 0, 1) x (1, 0, 0) in component "end v6 (1)"
mirror "Mirror2'" about plane through (0, 5, 0) normal (0, 0, 1) of 13 faces at (3.5, 2.5, -16.5) (4.5, 3.4925, -19.6247) (5.5, 4, -16.8333) (-4.5, 3.5474, -19.5738) (-6.5, 2.5, -16.1667) (-5.5, 4, -16.8333) (1.1667, 7.3333, -16) (6.5, 2.5, -16.1667) (2.1667, 9, -15.3333) (5.5, 1, -16.5) (-3.5, 2.5, -16.5) (5.5, 2.4004, -19.495) (-5.5, 2.4004, -19.495) on bodies 8 in component "end v6 (1)"
sketch "Sketch4 (8)" plane through (0, 0, 15) normal (0, 0, 1) x (1, 0, 0) in component "end v6 (1)"
  line L0 (6.5, 9) -> (6.5, 1)
  line L1 (6.5, 1) -> (-6.5, 1)
  line L2 (-6.5, 1) -> (-6.5, 9)
  line L3 (-6.5, 9) -> (6.5, 9)
  line L4 (-7.5, 0) -> (7.5, 0)
  line L5 (7.5, 0) -> (7.5, 10)
  line L6 (7.5, 10) -> (-7.5, 10)
  line L7 (-7.5, 10) -> (-7.5, 0)
sketch "Sketch5 (8)" plane through (6.5, 0, 0) normal (1, 0, 0) x (0, 0, -1) in component "end v6 (1)"
  circle A0 centre (-18.5, 2.5) radius 1
  line L0 (-16, 9) -> (-16, 4)
  line L1 (-16, 4) -> (-18.5, 4)
  arc A1 (-18.5, 4) -> (-18.5, 1) centre (-18.5, 2.5) ccw
  line L2 (-18.5, 1) -> (-15, 1)
  line L3 (-15, 1) -> (-15, 9)
  line L4 (-15, 9) -> (-16, 9)
sketch "Sketch6 (7)" plane through (0, 0, 16) normal (0, 0, 1) x (1, 0, 0) in component "end v6 (1)"
  line L0 (-3.5, 4) -> (-3.5, 1)
  line L1 (-3.5, 1) -> (3.5, 1)
  line L2 (3.5, 1) -> (3.5, 4)
  line L3 (3.5, 4) -> (6.5, 4)
  line L4 (6.5, 4) -> (6.5, 9)
  line L5 (6.5, 9) -> (-6.5, 9)
  line L6 (-6.5, 9) -> (-6.5, 4)
  line L7 (-6.5, 4) -> (-3.5, 4)
fillet "Fillet1''" radius 3 1 edges at (0, 0, 15) on bodies 8 in component "end v6 (1)"
sketch "Sketch1 (9)" plane through (0, 0, 0) normal (1, 0, 0) x (0, 0, -1) in component "turner v14 (1)"
  line L0 (10, -10) -> (-10, -10)
  line L1 (-10, -10) -> (-10, 10)
  line L2 (-10, 10) -> (10, 10)
  line L3 (10, 10) -> (10, -10)
  line L4 (10, -10) -> (-10, 10) construction
  line L5 (-10, -10) -> (10, 10) construction
  dimension "d4_8" = 20
  dimension "d5_11" = 20
  constraint horizontal L0
  constraint perpendicular L0 L1
  constraint parallel L0 L2
  constraint parallel L1 L3
  constraint coincident L4 origin
  constraint coincident L5 origin
  measures "d4_8" distance of L0.start L2.end
  measures "d5_11" distance of L0.start L0.end
extrude "Extrude1''''''''" add sketch "Sketch1 (9)" along normal blind 20 separate body makes body 9 in component "turner v14 (1)"
sketch "Sketch2 (9)" plane through (0, 0, -10) normal (0, 0, -1) x (-1, 0, 0) in component "turner v14 (1)"
  line L0 (0, -10) -> (0, 10)
  line L1 (0, 10) -> (-20, 10)
  line L2 (-20, 10) -> (-20, -10)
  line L3 (-20, -10) -> (0, -10)
  line L4 (-10, 10) -> (-3.5, 10)
  line L5 (-3.5, 10) -> (-3.5, 3.5)
  line L6 (-10, 10) -> (-10, 4.4853) construction
  line L7 (-10, 10) -> (-16.5, 10)
  line L8 (-16.5, 10) -> (-16.5, 3.5)
  arc A0 (-16.5, 3.5) -> (-3.5, 3.5) centre (-10, 3.5) ccw
  dimension "d12_7" = 6.5
  dimension "d13_7" = 6.5
  constraint midpoint L1 L4.start
  constraint parallel L1 L4
  constraint perpendicular L4 L5
  constraint perpendicular L1 L6
  constraint symmetric L4.start L6 L7.start
  constraint symmetric L4.end L6 L7.end
  constraint symmetric L5.end L6 L8.end
  constraint tangent L5 A0
  measures "d12_7" distance of L4.start L4.end
  measures "d13_7" distance of L4.end L5.end
extrude "Extrude2''''''''" cut sketch "Sketch2 (9)" against normal blind 10 contours L1 L4 L5 L7 L8 A0 bodies 9 in component "turner v14 (1)"
sketch "Sketch3 (9)" plane through (3.5, 0, 0) normal (1, 0, 0) x (0, 0, -1) in component "turner v14 (1)"
  line L0 (10, 3.5) -> (10, 10)
  line L1 (10, 10) -> (0, 10)
  line L2 (0, 10) -> (0, 3.5)
  line L3 (0, 3.5) -> (10, 3.5)
  line L4 (5, 3.5) -> (5, 7.5) construction
  circle A0 centre (5, 7.5) radius 1
  dimension "d20_8" = 4
  dimension "d22_8" = 5
  dimension "d23_4" = 2
  constraint coincident L3 L4.start
  constraint perpendicular L3 L4
  constraint coincident L4.end A0.centre
  measures "d20_8" distance of L4.start L4.end
  measures "d22_8" distance of L0 L4
  measures "d23_4" diameter of A0
extrude "Extrude3''''''''" add sketch "Sketch3 (9)" along normal up to surface (13 mm away) contours A0 bodies 9 in component "turner v14 (1)"
sketch "Sketch4 (9)" plane through (0, 0, 10) normal (0, 0, 1) x (1, 0, 0) in component "turner v14 (1)"
  line L0 (0, 10) -> (0, -10)
  line L1 (0, -10) -> (20, -10)
  line L2 (20, -10) -> (20, 10)
  line L3 (20, 10) -> (0, 10)
sketch "Sketch5 (9)" plane through (0, 0, 10) normal (0, 0, 1) x (1, 0, 0) in component "turner v14 (1)"
  circle A0 centre (10, 0) radius 1.5
  line L0 (20, 10) -> (0, 10)
  line L1 (20, -10) -> (20, 10)
  dimension "d28_7" = 3
  dimension "d29_10" = 10
  dimension "d30_8" = 10
  measures "d28_7" diameter of A0
  measures "d29_10" distance of A0.centre L0
  measures "d30_8" distance of A0.centre L1
extrude "Extrude4''''" add sketch "Sketch5 (9)" along normal blind 3 bodies 9 in component "turner v14 (1)"
fillet "Fillet1'''" radius 7 1 edges at (10, -10, -10) on bodies 9 in component "turner v14 (1)"
fillet "Fillet2'" radius 7 3 edges at (20, -10, 3.5) (20, -7.9497, -7.9497) (20, 3.5, -10) on bodies 9 in component "turner v14 (1)"
fillet "Fillet3'" radius 7 3 edges at (0, 3.5, -10) (0, -7.9497, -7.9497) (0, -10, 3.5) on bodies 9 in component "turner v14 (1)"
sketch "Sketch1 (10)" plane through (0, 0, 0) normal (1, 0, 0) x (0, 0, -1) in component "top v5 (2)"
  line L0 (0, 0) -> (20, 0)
  line L1 (20, 0) -> (20, 10)
  line L2 (20, 10) -> (0, 3)
  line L3 (0, 3) -> (0, 0)
  dimension "d5_13" = 20
  dimension "d6_11" = 10
  dimension "d7_11" = 3
  constraint coincident L0.start L3.end
  constraint horizontal L0
  constraint perpendicular L0 L1
  constraint perpendicular L0 L3
  measures "d5_13" distance of L0.start L0.end
  measures "d6_11" distance of L0.end L1.end
  measures "d7_11" distance of L2.end L0.start
extrude "Extrude1'''''''''" add sketch "Sketch1 (10)" along normal blind 15 separate body makes body 10 in component "top v5 (2)"
sketch "Sketch2 (10)" plane through (15, 0, 0) normal (1, 0, 0) x (0, 0, -1) in component "top v5 (2)"
  line L0 (0, 3) -> (0, 0)
  line L1 (0, 0) -> (20, 0)
  line L2 (20, 0) -> (20, 10)
  line L3 (20, 10) -> (0, 3)
ref_plane "WorkPlane1" through (7.5, 5, -21) normal (0, 0, -1) x (0, 1, 0) in component "top v5 (2)"
sketch "Sketch3 (10)" plane through (7.5, 5, -21) normal (0, 0, -1) x (1, 0, 0) in component "top v5 (2)"
  line L0 (-6.5, 4) -> (6.5, 4)
  line L1 (6.5, 4) -> (6.5, -4)
  line L2 (6.5, -4) -> (-6.5, -4)
  line L3 (-6.5, -4) -> (-6.5, 4)
  line L4 (-6.5, 4) -> (6.5, -4) construction
  line L5 (6.5, 4) -> (-6.5, -4) construction
  dimension "d17_6" = 13
  dimension "d18_8" = 8
  constraint horizontal L0
  constraint perpendicular L0 L1
  constraint parallel L0 L2
  constraint parallel L1 L3
  constraint coincident L4 origin
  constraint coincident L5 origin
  measures "d17_6" distance of L1.end L2.end
  measures "d18_8" distance of L0.start L2.end
extrude "Extrude2'''''''''" add sketch "Sketch3 (10)" against normal blind 1 bodies 10 in component "top v5 (2)"